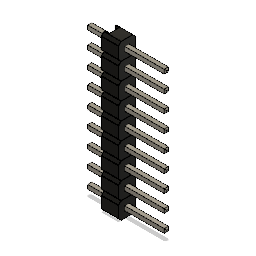
pinsStraightMale (Autodesk Fusion 360 design; units mm, degrees)
Autodesk Fusion 360 part; units mm, degrees
sketch "Sketch1" plane through (0, 0, 0) normal (0, 1, 0) x (1, 0, 0) in component "Pin"
  line L0 (0, 0) -> (11.684, 0)
  line L1 (11.684, 0) -> (11.684, -0.635)
  line L2 (11.684, -0.635) -> (0, -0.635)
  line L3 (0, -0.635) -> (0, 0)
  dimension "d2" = 0.635
  dimension "d3" = 11.684
  measures "d3" distance of L0.start
extrude "Extrude1" add sketch "Sketch1" along normal blind 0.635 makes body 1 in component "Pin"
chamfer "Chamfer1" distance 0.1905 angle 45 8 edges at (0, 0.3175, 0.635) (0, 0.635, 0.3175) (0, 0.3175, 0) (0, 0, 0.3175) (11.684, 0.635, 0.3175) (11.684, 0.3175, 0) (11.684, 0, 0.3175) (11.684, 0.3175, 0.635) on bodies 1 in component "Pin"
sketch "Sketch1 (2)" plane through (0, 0, 0) normal (0, 1, 0) x (1, 0, 0) in component "Plastic"
  line L0 (0, -0.4445) -> (0, -0.1905)
  line L1 (0, -0.3175) -> (3.81, -0.3175)
  line L2 (3.81, -1.0795) -> (3.81, 0.4445)
  line L3 (0.1905, 0) -> (11.4935, 0) construction
  line L4 (3.81, 0.4445) -> (3.81, 0.9525) construction
  line L5 (3.81, -1.0795) -> (3.81, -1.5875) construction
  line L6 (3.81, 0.4445) -> (3.175, 0.4445)
  line L7 (3.81, -1.0795) -> (3.175, -1.0795)
  line L8 (3.175, -1.0795) -> (3.175, -1.5875)
  line L9 (3.175, 0.4445) -> (3.175, 0.9525)
  line L10 (3.175, 0.9525) -> (5.715, 0.9525)
  line L11 (5.715, 0.9525) -> (5.715, -1.5875)
  line L12 (3.175, -1.5875) -> (5.715, -1.5875)
  dimension "d7" = 3.81
  dimension "d8" = 1.524
  dimension "d9" = 0.508
  dimension "d11" = 0.635
  dimension "d12" = 2.54
  measures "d7" distance of origin
extrude "Extrude1'" add sketch "Sketch1 (2)" along normal mid plane 2.54 from surface at 0.3175 separate body makes body 2 in component "Plastic"
chamfer "Chamfer1'" distance 0.4 angle 45 4 edges at (4.445, 1.5875, -0.9525) (4.445, -0.9525, -0.9525) (4.445, 1.5875, 1.5875) (4.445, -0.9525, 1.5875) on bodies 2 in component "Plastic"
sketch "Sketch1 (3)" plane through (0, 0, 0) normal (0, 0, 1) x (1, 0, 0)
  line L0 (0, 0.1905) -> (0, 0.4445)
  line L1 (0, 0.3175) -> (0, 14)
other "PathPattern1" in component "Header"
component "Header" placed x (1, 0, 0) y (0, 1, 0) z (0, 0, 1) at (0, 0, 0)
component "Header" placed x (1, 0, 0) y (0, 1, 0) z (0, 0, 1) at (0, 2.54, 0)
component "Header" placed x (1, 0, 0) y (0, 1, 0) z (0, 0, 1) at (0, 5.08, 0)
component "Header" placed x (1, 0, 0) y (0, 1, 0) z (0, 0, 1) at (0, 7.62, 0)
component "Header" placed x (1, 0, 0) y (0, 1, 0) z (0, 0, 1) at (0, 10.16, 0)
component "Header" placed x (1, 0, 0) y (0, 1, 0) z (0, 0, 1) at (0, 12.7, 0)
component "Header" placed x (1, 0, 0) y (0, 1, 0) z (0, 0, 1) at (0, 15.24, 0)
component "Header" placed x (1, 0, 0) y (0, 1, 0) z (0, 0, 1) at (0, 17.78, 0)
component "Header" placed x (1, 0, 0) y (0, 1, 0) z (0, 0, 1) at (0, 20.32, 0)
component "Pin" placed x (1, 0, 0) y (0, 1, 0) z (0, 0, 1) at (0, 0, 0) in component "Header"
component "Plastic" placed x (1, 0, 0) y (0, 1, 0) z (0, 0, 1) at (0, 0, 0) in component "Header"
equation "pinCount = 9"
equation "d13 = 0.025 in / 2"
equation "d19 = pinCount"
equation "d21 = pinCount"
